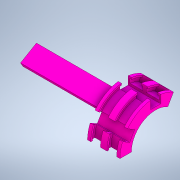
# Autodesk Inventor part: buttons_base
Saved by Autodesk Inventor 2020 (Build 240168000, 168)
## iProperties
Created: 2019-11-15
Part Number: buttons_base
Material: Generic
Document SubType Name: Modeling
Designer: suchanek
Density: 1 g/cm^3
Appearance: Default
Author: suchanek
Autodesk Inventor part; units mm, degrees
ref_plane "YZ Plane" through (0, 0, 0) normal (1, 0, 0) x (0, 1, 0)
ref_plane "XZ Plane" through (0, 0, 0) normal (0, 1, 0) x (-1, 0, 0)
ref_plane "XY Plane" through (0, 0, 0) normal (0, 0, 1) x (1, 0, 0)
sketch "Sketch1" plane through (0, 0, 0) normal (1, 0, 0) x (0, 1, 0)
  arc A0 (12.9904, -7.5) -> (0, 15) centre (0, 0) ccw
  line L0 (0, 15) -> (0, 22)
  arc A1 (19.0526, -11) -> (0, 22) centre (0, 0) ccw
  line L1 (0, 0) -> (19.0526, -11) construction
  line L2 (0, 0) -> (0, 22) construction
  line L3 (12.9904, -7.5) -> (19.0526, -11)
  dimension "d0" = 15
  dimension "d1" = 7
  dimension "d2" = 120
  constraints: 8 end point, 4 point on circle, 2 centre point, 2 coincident, 2 line through centre, 1 vertical
  measures "d0" radius of A0
  measures "d1" distance of L0.start L0.end
  measures "d2" angle of L1 L2
extrude "Extrusion1" add sketch "Sketch1" along normal blind 20
sketch "Sketch2" plane through (20, 0, 0) normal (1, 0, 0) x (0, 0, -1)
  arc A0 (8.5, 14.7224) -> (-17, 0) centre (0, 0) ccw
  line L0 (-16.0256, 5.6728) -> (-12.9256, 11.0422)
  line L1 (-12.9256, 11.0422) -> (-21.5858, 16.0422)
  line L2 (-21.5858, 16.0422) -> (-24.6858, 10.6728)
  line L3 (-24.6858, 10.6728) -> (-16.0256, 5.6728)
  line L4 (-3.1, 16.715) -> (3.1, 16.715)
  line L5 (3.1, 16.715) -> (3.1, 26.715)
  line L6 (3.1, 26.715) -> (-3.1, 26.715)
  line L7 (-3.1, 26.715) -> (-3.1, 16.715)
  line L8 (0, 0) -> (-2.9003, 5.0235)
  line L9 (7.5, 12.9904) -> (11, 19.0526) projected
  line L10 (-22, 0) -> (-15, 0) projected
  line L11 (0, 0) -> (0, 12.1585)
  dimension "d5" = 6.2
  dimension "d6" = 17
  dimension "d7" = 10
  constraints: 20 end point, 6 point on circle, 5 parallel, 3 symmetric about line, 2 perpendicular, 2 point on line, 1 centre point, 1 coincident, 1 other
  measures "d5" distance of L5.end L6.end
  measures "d6" radius of A0
  measures "d7" distance of L6.end L4.start
extrude "Extrusion2" cut sketch "Sketch2" against normal blind 20
sketch "Sketch3" plane through (0, 0, 15) normal (0, -1, 0) x (1, 0, 0)
  line L0 (0, 7) -> (20, 7) projected
  line L1 (2, 7) -> (8, 7)
  line L2 (8, 7) -> (8, 6)
  line L3 (8, 6) -> (2, 6)
  line L4 (2, 6) -> (2, 7)
  line L5 (1, 6) -> (9, 6)
  line L6 (9, 6) -> (9, 3.5)
  line L7 (9, 3.5) -> (1, 3.5)
  line L8 (1, 3.5) -> (1, 6)
  line L9 (10, 7) -> (10, 5.9883)
  line L10 (18, 7) -> (12, 7)
  line L11 (12, 7) -> (12, 6)
  line L12 (12, 6) -> (18, 6)
  line L13 (18, 6) -> (18, 7)
  line L14 (19, 6) -> (11, 6)
  line L15 (11, 6) -> (11, 3.5)
  line L16 (11, 3.5) -> (19, 3.5)
  line L17 (19, 3.5) -> (19, 6)
  line L18 (0, 7) -> (0, 0) projected
  line L19 (0, -15) -> (33.934, -15)
  point P0 (18, 7)
  dimension "d10" = 10
  dimension "d11" = 1
  dimension "d12" = 1
  dimension "d13" = 1
  dimension "d14" = 1
  dimension "d15" = 1
  dimension "d16" = 2.5
  constraints: 36 end point, 8 symmetric about line, 4 parallel, 3 horizontal, 3 point on line, 2 perpendicular, 1 midpoint, 1 vertical
  measures "d10" distance from line of L0.end L9
  measures "d11" distance between parallel lines of L9 L6
  measures "d12" distance between parallel lines of L18 L8
  measures "d13" distance between parallel lines of L8 L4
  measures "d14" distance between parallel lines of L6 L2
  measures "d15" distance of L3.end L1.start
  measures "d16" distance of L7.end L5.start
revolve "Revolution1" cut sketch "Sketch3" angle 118 about axis through (0, 0, 0) along (-1, 0, 0)
sketch "Sketch4" plane through (0, 0, 0) normal (-1, 0, 0) x (0, 0, 1)
  arc A0 (15, 0) -> (-7.5, 12.9904) centre (0, 0) ccw projected
  arc A1 (15, 0) -> (-7.5, 12.9904) centre (0, 0) ccw
  line L0 (2.0302, 14.862) -> (3.5302, 17.4601)
  line L1 (3.5302, 17.4601) -> (13.3558, 11.7873)
  line L2 (13.3558, 11.7873) -> (11.8558, 9.1892)
  line L3 (22, 0) -> (15, 0) projected
  line L4 (-7.5, 12.9904) -> (15, 0)
  line L5 (12.9256, 11.0422) -> (16.0256, 5.6728) projected
  line L6 (16.0256, 5.6728) -> (12.9313, 11.0323)
  line L7 (12.9313, 11.0323) -> (13.7973, 11.5323)
  line L8 (13.7973, 11.5323) -> (16.8916, 6.1728)
  line L9 (16.8916, 6.1728) -> (16.0256, 5.6728)
  line L10 (-3.1, 16.715) -> (3.1, 16.715) projected
  line L11 (-3.1, 16.715) -> (3.0887, 16.715)
  line L12 (3.0887, 16.715) -> (3.0887, 17.715)
  line L13 (3.0887, 17.715) -> (-3.1, 17.715)
  line L14 (-3.1, 17.715) -> (-3.1, 16.715)
  dimension "d18" = 3
  dimension "d21" = 1
  dimension "d22" = 1
  dimension "d23" = 12.3652
  constraints: 24 end point, 5 parallel, 4 perpendicular, 4 point on circle, 4 point on line, 2 collinear, 1 centre point, 1 coincident
  measures "d18" distance of L1.end L2.end
  measures "d21" distance of L6.end L7.end
  measures "d22" distance of L12.end L11.end
  measures "d23" distance of L7.end L12.end
extrude "Extrusion3" add sketch "Sketch4" along normal blind 50 contours A0 L0 L1 L2
body "Solid1"
